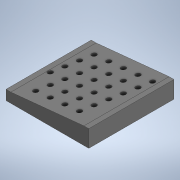
# Autodesk Inventor part: FiberJig
Saved by Autodesk Inventor 2021.1 (Build 251245010, 245A)
## iProperties
Created: 2021-07-07
Part Number: FiberJig
Material: Generic
Document SubType Name: Modeling
Designer: jloeb
Density: 1 g/cm^3
Appearance: Default
Author: jloeb
Autodesk Inventor part; units mm, degrees
ref_plane "YZ Plane" through (0, 0, 0) normal (1, 0, 0) x (0, 1, 0)
sketch "Sketch1" plane through (0, 0, 0) normal (0, 0, 1) x (1, 0, 0)
  line L0 (0, 0) -> (30, 0)
  line L1 (30, 0) -> (30, 3)
  line L2 (30, 3) -> (0, 0)
  dimension "d0" = 30
  dimension "d1" = 3
  constraints: 6 end point, 1 horizontal, 1 vertical
  measures "d0" distance of L0.start L0.end
  measures "d1" distance of L0.end L1.end
extrude "Extrusion1" add sketch "Sketch1" along normal blind 35
sketch "Sketch2" plane through (0, 0, 0) normal (0, -1, 0) x (1, 0, 0)
  circle A0 centre (26.2, 15) radius 0.6
  line L0 (0, 35) -> (30, 35) projected
  line L1 (30, 0) -> (30, 35) projected
  circle A1 centre (20.2, 15) radius 0.6
  circle A2 centre (14.2, 15) radius 0.6
  circle A3 centre (8.2, 15) radius 0.6
  circle A4 centre (2.2, 15) radius 0.6
  circle A5 centre (27.2, 10) radius 0.6
  circle A6 centre (21.2, 10) radius 0.6
  circle A7 centre (15.2, 10) radius 0.6
  circle A8 centre (9.2, 10) radius 0.6
  circle A9 centre (3.2, 10) radius 0.6
  circle A10 centre (28.2, 5) radius 0.6
  circle A11 centre (22.2, 5) radius 0.6
  circle A12 centre (16.2, 5) radius 0.6
  circle A13 centre (10.2, 5) radius 0.6
  circle A14 centre (4.2, 5) radius 0.6
  line L2 (0, 0) -> (30, 0) projected
  circle A15 centre (25.2, 20) radius 0.6
  circle A16 centre (19.2, 20) radius 0.6
  circle A17 centre (13.2, 20) radius 0.6
  circle A18 centre (7.2, 20) radius 0.6
  circle A19 centre (1.2, 20) radius 0.6
  circle A20 centre (24.2, 25) radius 0.6
  circle A21 centre (18.2, 25) radius 0.6
  circle A22 centre (12.2, 25) radius 0.6
  circle A23 centre (6.2, 25) radius 0.6
  circle A24 centre (23.2, 30) radius 0.6
  circle A25 centre (17.2, 30) radius 0.6
  circle A26 centre (11.2, 30) radius 0.6
  circle A27 centre (5.2, 30) radius 0.6
  dimension "d4" = 1.2
  dimension "d6" = 3.8
  dimension "d9" = 6
  dimension "d14" = 1.2
  dimension "d16" = 1
  dimension "d17" = 5
  dimension "d20" = 6
  dimension "d25" = 1.2
  dimension "d26" = 1
  dimension "d27" = 5
  dimension "d30" = 6
  dimension "d87" = 5
  dimension "d88" = 1.2
  dimension "d89" = 5
  dimension "d90" = 1
  dimension "d93" = 6
  dimension "d109" = 1.2
  dimension "d110" = 5
  dimension "d111" = 1
  dimension "d114" = 6
  dimension "d119" = 1.2
  dimension "d120" = 1
  dimension "d121" = 5
  dimension "d124" = 6
  constraints: 28 centre point, 6 horizontal, 44 other
  measures "d4" diameter of A0
  measures "d6" distance from line of L1 A0.centre
  measures "d9" distance of A0.centre A1.centre
  measures "d14" diameter of A5
  measures "d16" horizontal distance of A5.centre A0.centre
  measures "d17" vertical distance of A0.centre A5.centre
  measures "d20" distance of A5.centre A6.centre
  measures "d25" diameter of A10
  measures "d26" horizontal distance of A5.centre A10.centre
  measures "d27" vertical distance of A10.centre A5.centre
  measures "d30" distance of A10.centre A11.centre
  measures "d87" distance from line of L2 A10.centre
  measures "d88" diameter of A15
  measures "d89" vertical distance of A0.centre A15.centre
  measures "d90" horizontal distance of A0.centre A15.centre
  measures "d93" distance of A15.centre A16.centre
  measures "d109" diameter of A20
  measures "d110" vertical distance of A15.centre A20.centre
  measures "d111" horizontal distance of A15.centre A20.centre
  measures "d114" distance of A20.centre A21.centre
  measures "d119" diameter of A24
  measures "d120" horizontal distance of A20.centre A24.centre
  measures "d121" vertical distance of A24.centre A20.centre
  measures "d124" distance of A24.centre A25.centre
extrude "Extrusion2" cut sketch "Sketch2" against normal through all
sketch "Sketch4" plane through (0, 0, 35) normal (0, 0, 1) x (1, 0, 0)
  line L0 (30, 3) -> (0, 0) projected
  line L1 (0, 0) -> (0, 4)
  line L2 (30, 0) -> (30, 3) projected
  line L3 (30, 3) -> (30, 7)
  line L4 (30, 7) -> (0, 4)
  line L5 (0, 0) -> (30, 3)
  dimension "d41" = 4
  dimension "d42" = 4
  constraints: 8 end point, 2 vertical
  measures "d41" distance of L0.end L1.end
  measures "d42" distance of L0.start L3.end
extrude "Extrusion4" add sketch "Sketch4" against normal blind 35
sketch "Sketch5" plane through (30, 0, 35) normal (1, 0, 0) x (0, 0, -1)
  line L0 (0, 7) -> (0, 4) projected
  line L1 (35, 0) -> (0, 0)
  line L2 (0, 0) -> (0, 7)
  line L3 (0, 7) -> (35, 7)
  line L4 (35, 7) -> (35, 0)
  constraints: 8 end point, 2 parallel, 1 horizontal, 1 perpendicular
extrude "Extrusion5" add sketch "Sketch5" along normal blind 2
sketch "Sketch7" plane through (0, 0, 35) normal (-1, 0, 0) x (0, 0, 1)
  line L0 (0, 7) -> (0, 4) projected
  line L1 (0, 4) -> (-35, 4)
  line L2 (-35, 4) -> (-35, 0)
  line L3 (-35, 0) -> (0, 0)
  line L4 (0, 0) -> (0, 4)
  constraints: 8 end point, 2 parallel, 1 horizontal, 1 perpendicular
extrude "Extrusion6" add sketch "Sketch7" along normal blind 2
ref_plane "Work Plane2" through (0, 7, 0) normal (0, -1, 0) x (1, 0, 0)
sketch "Sketch6" plane through (0, 7, 0) normal (0, -1, 0) x (1, 0, 0)
  circle A0 centre (26.2, 15) radius 1
  line L0 (0, 0) -> (30, 0) projected
  line L1 (30, 35) -> (30, 0) projected
  line L2 (30, 35) -> (0, 35) projected
  circle A1 centre (20.2, 15) radius 1
  circle A2 centre (14.2, 15) radius 1
  circle A3 centre (8.2, 15) radius 1
  circle A4 centre (2.2, 15) radius 1
  circle A5 centre (27.2, 10) radius 1
  circle A6 centre (21.2, 10) radius 1
  circle A7 centre (15.2, 10) radius 1
  circle A8 centre (9.2, 10) radius 1
  circle A9 centre (3.2, 10) radius 1
  circle A10 centre (28.2, 5) radius 1
  circle A11 centre (22.2, 5) radius 1
  circle A12 centre (16.2, 5) radius 1
  circle A13 centre (10.2, 5) radius 1
  circle A14 centre (4.2, 5) radius 1
  circle A15 centre (25.2, 20) radius 1
  circle A16 centre (19.2, 20) radius 1
  circle A17 centre (13.2, 20) radius 1
  circle A18 centre (7.2, 20) radius 1
  circle A19 centre (1.2, 20) radius 1
  circle A20 centre (24.2, 25) radius 1
  circle A21 centre (18.2, 25) radius 1
  circle A22 centre (12.2, 25) radius 1
  circle A23 centre (6.2, 25) radius 1
  circle A24 centre (23.2, 30) radius 1
  circle A25 centre (17.2, 30) radius 1
  circle A26 centre (11.2, 30) radius 1
  circle A27 centre (5.2, 30) radius 1
  dimension "d49" = 2
  dimension "d52" = 3.8
  dimension "d60" = 6
  dimension "d65" = 2
  dimension "d66" = 5
  dimension "d67" = 1
  dimension "d70" = 6
  dimension "d75" = 2
  dimension "d76" = 5
  dimension "d77" = 1
  dimension "d80" = 6
  dimension "d98" = 5
  dimension "d99" = 2
  dimension "d100" = 5
  dimension "d101" = 1
  dimension "d104" = 6
  dimension "d129" = 2
  dimension "d130" = 5
  dimension "d131" = 1
  dimension "d134" = 6
  dimension "d139" = 2
  dimension "d140" = 5
  dimension "d141" = 1
  dimension "d144" = 6
  constraints: 28 centre point, 6 horizontal, 44 other
  measures "d49" diameter of A0
  measures "d52" distance from line of L1 A0.centre
  measures "d60" distance of A0.centre A1.centre
  measures "d65" diameter of A5
  measures "d66" vertical distance of A0.centre A5.centre
  measures "d67" horizontal distance of A0.centre A5.centre
  measures "d70" distance of A5.centre A6.centre
  measures "d75" diameter of A10
  measures "d76" vertical distance of A5.centre A10.centre
  measures "d77" horizontal distance of A5.centre A10.centre
  measures "d80" distance of A10.centre A11.centre
  measures "d98" distance from line of L0 A10.centre
  measures "d99" diameter of A15
  measures "d100" vertical distance of A0.centre A15.centre
  measures "d101" horizontal distance of A0.centre A15.centre
  measures "d104" distance of A15.centre A16.centre
  measures "d129" diameter of A20
  measures "d130" vertical distance of A15.centre A20.centre
  measures "d131" horizontal distance of A15.centre A20.centre
  measures "d134" distance of A20.centre A21.centre
  measures "d139" diameter of A24
  measures "d140" vertical distance of A20.centre A24.centre
  measures "d141" horizontal distance of A24.centre A20.centre
  measures "d144" distance of A24.centre A25.centre
ref_plane "Work Plane3" through (0.398, 0.0199, 35) normal (-0.0995, 0.995, 0) x (0.995, 0.0995, 0)
extrude "Extrusion7" cut sketch "Sketch6" along normal up to surface surface through (0.398, 0.0199, 35) normal (-0.0995, 0.995, 0)
body "Solid1"
